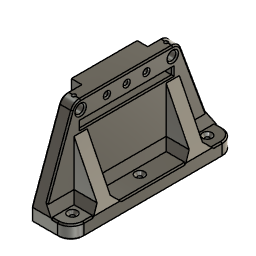
Backstop v11 (Autodesk Fusion 360 design; units mm, degrees)
Autodesk Fusion 360 part; units mm, degrees
sketch "Sketch1" plane through (0, 0, 0) normal (1, 0, 0) x (0, 1, 0)
  circle A0 centre (0, 0) radius 3.35
  circle A1 centre (70, 0) radius 3.35
  circle A2 centre (0, 0) radius 7
  circle A3 centre (70, 0) radius 7
  line L0 (70, 0) -> (70, -65) construction
  line L1 (7, 0) -> (7, -10)
  line L2 (70, -65) -> (-73.8132, -65) construction
  line L3 (63, 0) -> (63, -10)
  line L4 (-27.4676, -55) -> (97.4676, -55)
  line L5 (-6.5778, 2.3941) -> (-27.4676, -55)
  line L6 (0, 0) -> (70, 0) construction
  line L7 (35, 0) -> (35, -33.7499) construction
  line L8 (76.5778, 2.3941) -> (97.4676, -55)
  circle A4 centre (35, -10) radius 28 construction
  line L9 (-27.4676, -55) -> (-27.4676, -65)
  line L10 (97.4676, -55) -> (97.4676, -65)
  line L11 (97.4676, -65) -> (-27.4676, -65)
  line L12 (0, 7) -> (70, 7)
  dimension "d1" = 6.7
  dimension "d2" = 6.7
  dimension "d3" = 70
  dimension "d4" = 14
  dimension "d5" = 14
  dimension "d6" = 65
  dimension "d7" = 10
  dimension "d8" = 10
  dimension "d9" = 10
  dimension "d10" = 70
  dimension "d11" = 10
  constraint coincident A0.centre A2.centre
  constraint horizontal A0.centre A1.centre
  constraint concentric A0 A2
  constraint concentric A1 A3
  constraint coincident A1.centre A3.centre
  constraint vertical L0
  constraint coincident A2 L1.start
  constraint tangent A2 L1
  constraint vertical L1
  constraint horizontal L2
  constraint coincident A3 L3.start
  constraint vertical L3
  constraint tangent A3 L3
  constraint horizontal L4
  constraint coincident A2 L5.start
  constraint coincident L4 L5.end
  constraint tangent A2 L5
  constraint coincident L4.start L5.end
  constraint midpoint L6 L7.start
  constraint perpendicular L6 L7
  constraint symmetric L5.start L7 L8.start
  constraint symmetric L4.start L7 L4.end
  constraint coincident L4.end L8.end
  constraint tangent L3 A4
  constraint tangent L1 A4
  constraint horizontal L3.end A4.centre
  constraint coincident L2 L9.end
  constraint perpendicular L2 L9
  constraint perpendicular L4 L10
  constraint coincident A2 L12.start
  constraint coincident A3 L12.end
  constraint tangent A3 L12
  constraint tangent A2 L12
  measures "d1" diameter of A0
  measures "d2" diameter of A1
  measures "d3" distance of A0.centre A1.centre
  measures "d4" diameter of A2
  measures "d5" diameter of A3
  measures "d6" distance of A1.centre L0.end
  measures "d7" distance of L1.start L1.end
  measures "d8" distance of L3.start L3.end
  measures "d9" distance of L2 L4
  measures "d10" angle of L4 L5
  measures "d11" distance of L4.end L10.end
extrude "Extrude1" add sketch "Sketch1" against normal blind 10
extrude "Extrude2" add sketch "Sketch1" along normal blind 20 contours L4 L9 L10 L11
ref_plane "WorkPlane1" through (0, 35, -16.8749) normal (0, 1, 0) x (0, 0, -1)
ref_plane "WorkPlane2" through (0, 0, -16.8749) normal (0, 1, 0) x (0, 0, -1)
sketch "Sketch2" plane through (0, 0, 0) normal (0, 1, 0) x (1, 0, 0)
  line L0 (0, -2.3941) -> (0, 55)
  line L1 (0, 55) -> (20, 55)
  line L2 (0, 15) -> (20, 55)
  point P0 (0, 55)
  dimension "d18" = 20
  dimension "d19" = 40
  constraint coincident L0 L2.start
  constraint coincident L1 L2.end
  measures "d18" distance of P0 L1.end
  measures "d19" distance of L2.start P0
extrude "Extrude3" add sketch "Sketch2" along normal mid plane 10
mirror "Mirror1" about plane through (0, 35, -16.8749) normal (0, 1, 0) of "Extrude3"
sketch "Sketch3" plane through (0, 0, -55) normal (0, 0, 1) x (-1, 0, 0)
  line L0 (-20, -65) -> (0, -65)
  line L1 (0, -65) -> (0, -5)
  line L2 (0, -5) -> (-20, -5)
  line L3 (-20, -5) -> (-20, -65)
  line L4 (-10, -65) -> (-10, -5) construction
  line L5 (-20, -35) -> (0, -35) construction
  circle A0 centre (-10, -35) radius 1.6
  line L6 (-20, -97.4676) -> (-20, -75)
  line L7 (-20, 5) -> (-20, 27.4676)
  line L8 (-20, -86.2338) -> (-10, -86.2338) construction
  circle A1 centre (-10, -86.2338) radius 1.6
  circle A2 centre (-10, 16.2338) radius 1.6
  dimension "d24" = 3.2
  dimension "d25" = 3.2
  constraint midpoint L0 L4.start
  constraint midpoint L2 L4.end
  constraint midpoint L3 L5.start
  constraint midpoint L1 L5.end
  constraint midpoint L5 A0.centre
  constraint midpoint L6 L8.start
  constraint perpendicular L4 L8
  constraint vertical L4.start L8.end
  constraint coincident L8.end A1.centre
  constraint symmetric L5 A1 A2
  measures "d24" diameter of A0
  measures "d25" diameter of A1
extrude "Extrude4" cut sketch "Sketch3" against normal blind 40 contours A0 | A1 | A2
chamfer "Chamfer1" distance 2 angle 45 3 edges at (11.4917, -16.8124, -55) (11.4917, 34.4214, -55) (11.4917, 85.6552, -55)
sketch "Sketch5" plane through (-10, 0, 0) normal (-1, 0, 0) x (0, -1, 0)
  circle A0 centre (-70, 0) radius 3.35
  circle A1 centre (0, 0) radius 3.35
  line L0 (27.4676, -65) -> (27.4676, -55)
  line L1 (27.4676, -55) -> (6.5778, 2.3941)
  arc A2 (6.5778, 2.3941) -> (0, 7) centre (0, 0) ccw
  line L2 (0, 7) -> (-70, 7)
  arc A3 (-70, 7) -> (-76.5778, 2.3941) centre (-70, 0) ccw
  line L3 (-76.5778, 2.3941) -> (-97.4676, -55)
  line L4 (-97.4676, -55) -> (-97.4676, -65)
  line L5 (-97.4676, -65) -> (27.4676, -65)
  line L6 (-35, 7) -> (-35, -65) construction
  line L7 (-10, 7) -> (-60, 7)
  line L8 (-60, 7) -> (-60, -65)
  line L9 (-60, -65) -> (-10, -65)
  line L10 (-10, -65) -> (-10, 7)
  line L11 (-10, 7) -> (-60, -65) construction
  line L12 (-60, 7) -> (-10, -65) construction
  point P0 (-35, -29)
  dimension "d39" = 50
  dimension "d40" = 72
  constraint midpoint L2 L6.start
  constraint midpoint L5 L6.end
  constraint horizontal L7
  constraint perpendicular L7 L8
  constraint parallel L7 L9
  constraint parallel L8 L10
  constraint coincident L11 P0
  constraint coincident L12 P0
  constraint midpoint L6 P0
  measures "d39" distance of L8.end L9.end
  measures "d40" distance of L7.end L8.end
extrude "Extrude6" add sketch "Sketch5" along normal blind 8 contours L2 L5 L7 L8 L9 L10
sketch "Sketch6" plane through (-18, 0, 0) normal (-1, 0, 0) x (0, -1, 0)
  line L0 (-10, -65) -> (-10, 7)
  line L1 (-10, 7) -> (-60, 7)
  line L2 (-60, 7) -> (-60, -65)
  line L3 (-60, -65) -> (-10, -65)
  line L4 (-35, -65) -> (-35, 7) construction
  line L5 (-70, -7.5) -> (0, -7.5)
  line L6 (0, -7.5) -> (0, -12.5)
  line L7 (0, -12.5) -> (-70, -12.5)
  line L8 (-70, -12.5) -> (-70, -7.5)
  line L9 (-97.4676, -65) -> (-60, -65)
  dimension "d45" = 70
  dimension "d46" = 5
  dimension "d47" = 52.5
  constraint midpoint L3 L4.start
  constraint midpoint L1 L4.end
  constraint horizontal L5
  constraint vertical L6
  constraint horizontal L7
  constraint vertical L8
  constraint symmetric L4 L6 L8
  measures "d45" distance of L5.start L5.end
  measures "d46" distance of L5.start L7.end
  measures "d47" distance of L7.end L9
extrude "Extrude7" cut sketch "Sketch6" against normal blind 85 contours L0 L2 L5 L7 | L0 L5 L6 L7 | L2 L5 L7 L8
fillet "Fillet1" radius 10 2 edges at (20, -27.4676, -60) (20, 97.4676, -60)
chamfer "Chamfer3" distance 5 angle 45 8 edges at (0, -16.2338, -55) (0, 51.2338, -55) (10, -5, -55) (0, 35, -55) (10, 65, -55) (0, 86.2338, -55) (10, 75, -55) (10, 5, -55)
ref_plane "WorkPlane3" through (-7.0239, 70, 7) normal (0, 0, 1) x (0, -1, 0)
sketch "Sketch4" plane through (0, 0, 7) normal (0, 0, 1) x (1, 0, 0)
  line L0 (-1, 70) -> (-9, 70) construction
  circle A0 centre (-5, 70) radius 1.35
  line L1 (-10, 66.65) -> (-10, 73.35)
  line L2 (0, 73.35) -> (0, 66.65)
  dimension "d34" = 2.7
  constraint midpoint L0 A0.centre
  measures "d34" diameter of A0
extrude "Extrude5" cut sketch "Sketch4" against normal blind 7
mirror "Mirror2" about plane through (0, 35, -16.8749) normal (0, 1, 0) of "Extrude5"
chamfer "Chamfer4" distance 1 angle 45 38 edges at (-18, 35, -7.5) (-10, 65, -7.5) (-10, 70, -10) (-10, 65, -12.5) (-18, 35, -12.5) (-10, 5, -12.5) (-10, 5, -7.5) (-10, 0, -10) (0, -16.1128, -23.8029) (0, 86.1128, -23.8029) (0, 74.015, 5.7341) (0, 35, 7) (0, -4.015, 5.7341) (0, -3.1233, 1.2114) (0, 66.8767, 1.2114) (0, 70, -10) (0, 35, -7.5) (0, 35, -12.5) (0, 0, -10) (-18, 60, -0.25) (-18, 35, 7) (-18, 10, -0.25) (-18, 10, -38.75) (-18, 60, -38.75) (-18, 35, -65) (-10, -17.0227, -26.3029) (-10, -4.015, 5.7341) (-10, 5, 7) (-10, 65, 7) (-10, 74.015, 5.7341) (-10, 87.0227, -26.3029) (-10, -8.7338, -65) (-10, 78.7338, -65) (-10, -27.4676, -60) (-10, 97.4676, -60) (-14, 60, -65) (-10, -3.1233, -1.2114) (-10, 66.8767, -1.2114)
chamfer "Chamfer5" distance 1 angle 45 12 edges at (17.0711, -24.5387, -55) (7.5, -27.4676, -55) (20, -13.7338, -55) (20, 35, -55) (20, 83.7338, -55) (7.5, 97.4676, -55) (17.0711, 94.5387, -55) (20, 35, -65) (17.0711, 94.5387, -65) (0.5, 97.4676, -65) (0.5, -27.4676, -65) (17.0711, -24.5387, -65)
sketch "Sketch7" plane through (0, 0, 0) normal (1, 0, 0) x (0, 1, 0)
  circle A0 centre (70, 0) radius 4.35
  line L0 (94.5836, -50) -> (75.6382, 2.0521)
  arc A1 (75.6382, 2.0521) -> (70, 6) centre (70, 0) ccw
  line L1 (70, 6) -> (0, 6)
  arc A2 (0, 6) -> (-5.6382, 2.0521) centre (0, 0) ccw
  line L2 (-5.6382, 2.0521) -> (-24.5836, -50)
  line L3 (-24.5836, -50) -> (-5, -50)
  line L4 (-5, -50) -> (-5, -15)
  line L5 (-5, -15) -> (5, -15)
  line L6 (5, -15) -> (5, -50)
  line L7 (5, -50) -> (65, -50)
  line L8 (65, -50) -> (65, -15)
  line L9 (65, -15) -> (75, -15)
  line L10 (75, -15) -> (75, -50)
  line L11 (75, -50) -> (94.5836, -50)
  circle A3 centre (0, 0) radius 4.35
  line L12 (-1, -13.5) -> (-1, -6.5)
  line L13 (-1, -6.5) -> (71, -6.5)
  line L14 (71, -6.5) -> (71, -13.5)
  line L15 (71, -13.5) -> (-1, -13.5)
  line L16 (35, 6) -> (35, -6.5) construction
  circle A4 centre (35, -0.25) radius 1.7
  line L17 (35, -0.25) -> (20, -0.25) construction
  circle A5 centre (20, -0.25) radius 1.7
  circle A6 centre (50, -0.25) radius 1.7
  dimension "d52" = 3.4
  dimension "d53" = 3.4
  dimension "d54" = 15
  constraint midpoint L1 L16.start
  constraint midpoint L13 L16.end
  constraint midpoint L16 A4.centre
  constraint coincident A4.centre L17.start
  constraint perpendicular L16 L17
  constraint coincident L17.end A5.centre
  constraint symmetric L16 A5 A6
  measures "d52" diameter of A4
  measures "d53" diameter of A5
  measures "d54" distance of A4.centre L17.end
extrude "Extrude8" cut sketch "Sketch7" against normal blind 15 contours A4 | A5 | A6
chamfer "Chamfer6" distance 1 angle 45 3 edges at (0, 18.415, 0.3647) (0, 33.415, 0.3647) (0, 48.415, 0.3647)
